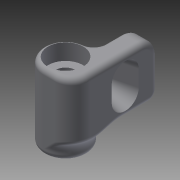
# Autodesk Inventor part: guia.tractora
Saved by Autodesk Inventor 2015 SP1 (Build 190203100, 203)
## iProperties
Created: 2015-07-01
Part Number: guia.tractora
Material: Generic
Document SubType Name: Modeling
Designer: pc
Density: 1 g/cm^3
Appearance: Default
Author: pc
Autodesk Inventor part; units mm, degrees
ref_plane "YZ Plane" through (0, 0, 0) normal (1, 0, 0) x (0, 1, 0)
ref_plane "XZ Plane" through (0, 0, 0) normal (0, 1, 0) x (-1, 0, 0)
ref_plane "XY Plane" through (0, 0, 0) normal (0, 0, 1) x (1, 0, 0)
sketch "Sketch10" plane through (0, 0, 0) normal (0, 0, 1) x (1, 0, 0)
  arc A0 (1.25, 3.7997) -> (0, -4) centre (0, 0) ccw
  line L0 (1.25, 3.7997) -> (1.25, 11.7997)
  line L1 (1.25, 11.7997) -> (5.25, 11.7997)
  line L2 (5.25, 11.7997) -> (5.25, -4)
  line L3 (5.25, -4) -> (0, -4)
  point P0 (1.25, -4)
  point P1 (1.25, -3)
  point P2 (3.25, 11.7997)
  dimension "d51" = 8
  dimension "d52" = 8
  dimension "d53" = 4
  dimension "d56" = 1.25
  constraints: 8 end point, 3 point on line, 2 perpendicular, 2 point on circle, 1 centre point, 1 coincident, 1 midpoint, 1 parallel, 1 tangent, 1 vertical
  measures "d51" diameter of A0
  measures "d52" distance of L0.start L0.end
  measures "d53" distance of L0.end L1.end
  measures "d56" distance from line of L0 point (0, 0)
extrude "Extrusion7" add sketch "Sketch10" along normal blind 10
sketch "Sketch15" plane through (0, 0, 0) normal (0, 0, -1) x (-1, 0, 0)
  arc A0 (0, -4) -> (-1.25, 3.7997) centre (0, 0) ccw projected
  circle A1 centre (0, 0) radius 4
  constraints: 1 centre point, 1 coincident, 1 concentric
extrude "Extrusion12" add sketch "Sketch15" along normal blind 4
sketch "Sketch16" plane through (0, 0, 10) normal (0, 0, 1) x (1, 0, 0)
  arc A0 (1.25, 3.7997) -> (0, -4) centre (0, 0) ccw projected
  circle A1 centre (0, 0) radius 3.25
  dimension "d71" = 6.5
  constraints: 1 centre point, 1 coincident
  measures "d71" diameter of A1
extrude "Extrusion13" cut sketch "Sketch16" against normal blind 3
sketch "Sketch17" plane through (0, 0, 7) normal (0, 0, 1) x (1, 0, 0)
  circle A0 centre (0, 0) radius 3.25 projected
  circle A1 centre (0, 0) radius 1.75
  dimension "d74" = 3.5
  constraints: 1 centre point, 1 coincident
  measures "d74" diameter of A1
extrude "Extrusion14" cut sketch "Sketch17" against normal through all contours A1
sketch "Sketch18" plane through (1.25, 3.7997, 0) normal (-1, 0, 0) x (0, 0, 1)
  line L0 (0, 8) -> (0, 0) projected
  line L1 (0, 0) -> (10, 0) projected
  line L2 (10, 8) -> (10, 0) projected
  line L3 (0, 8) -> (10, 8) projected
  line L4 (3.5, 2) -> (6.5, 2) construction
  line L5 (3.5, 0.5) -> (6.5, 0.5)
  line L6 (6.5, 3.5) -> (3.5, 3.5)
  arc A0 (3.5, 3.5) -> (3.5, 0.5) centre (3.5, 2) ccw
  arc A1 (6.5, 0.5) -> (6.5, 3.5) centre (6.5, 2) ccw
  point P0 (0, -3.7997)
  point P1 (5, 2)
  dimension "d77" = 3
  dimension "d78" = 3
  dimension "d79" = 6
  dimension "d80" = 5
  constraints: 8 end point, 4 point on circle, 4 tangent, 2 centre point, 1 horizontal, 1 midpoint, 1 parallel
  measures "d77" distance of L4.start L4.end
  measures "d78" diameter of A1
  measures "d79" distance from line of L3 point (5, 2)
  measures "d80" distance from line of L0 point (5, 2)
sketch "Sketch19" plane through (5.25, -4, 0) normal (1, 0, 0) x (0, 0, -1)
  line L0 (-10, 0) -> (-10, 15.7997) projected
  line L1 (0, 0) -> (0, 15.7997) projected
  line L2 (0, 15.7997) -> (-10, 15.7997) projected
  line L3 (-10, 0) -> (-10, 15.7997) projected
  line L4 (0, 0) -> (-10, 0) projected
  line L5 (0, 0) -> (-10, 0) projected
  line L6 (-10, 0) -> (-10, 15.7997) projected
  line L7 (-10, 15.7997) -> (0, 15.7997) projected
  line L8 (0, 15.7997) -> (0, 0) projected
  line L9 (0, 0) -> (-10, 0) projected
  line L10 (-10, 0) -> (-10, 15.7997) projected
  line L11 (-10, 15.7997) -> (0, 15.7997) projected
  line L12 (0, 15.7997) -> (0, 0) projected
  line L13 (-6.5, 11.2997) -> (-3.5, 11.2997) projected
  arc A0 (-6.5, 11.2997) -> (-6.5, 8.2997) centre (-6.5, 9.7997) ccw projected
  line L14 (-3.5, 8.2997) -> (-6.5, 8.2997) projected
  arc A1 (-3.5, 8.2997) -> (-3.5, 11.2997) centre (-3.5, 9.7997) ccw projected
  arc A2 (-6.5, 12.2997) -> (-6.5, 7.2997) centre (-6.5, 9.7997) ccw
  line L15 (-6.5, 12.2997) -> (-3.5, 12.2997)
  arc A3 (-3.5, 7.2997) -> (-3.5, 12.2997) centre (-3.5, 9.7997) ccw
  line L16 (-3.5, 7.2997) -> (-6.5, 7.2997)
  point P0 (0, 4)
  dimension "d90" = 1
  constraints: 4 end point, 4 point on circle, 2 centre point, 3 other
  measures "d90" radial gap between concentric circles of A0 A2
loft "Loft4" cut profiles "Sketch19", "Sketch18" contours L13 A1 L14 A0 | L15 A3 L16 A2 / A0 L6 A1 L5
fillet "Fillet5" radius 2.76 1 edges at (3.9496, -0.633, 0)
fillet "Fillet6" radius 2 2 edges at (1.25, 3.7997, 5) (1.25, 3.7997, -1.38)
fillet "Fillet7" radius 1.47 1 edges at (3.25, 11.7997, 0)
fillet "Fillet8" radius 2.81 1 edges at (3.25, 11.7997, 10)
fillet "Fillet9" radius 3.26 1 edges at (5.25, -4, 4.9977)
fillet "Fillet10" radius 1 20 edges at (5.25, 10.9766, 9.177) (5.25, 4.1248, 10) (4.2952, -3.0452, 10) (0.995, -4, 10) (-3.9921, -0.2505, 10) (0.75, 4.6301, 10) (1.25, 7.4713, 10) (1.25, 10.9766, 9.177) (1.25, 11.7997, 4.33) (1.25, 11.3691, 0.4306) (1.25, 8.4865, 0) (1.25, 6.2956, -0.0212) (0.4041, 4.3195, -1.4359) (5.25, 11.3691, 0.4306) (5.25, 7.2941, 0) (5.25, 1.7733, -0.2836) (4.2009, -3.1357, -0.4548) (1.6157, -4, -1.4815) (0.6194, -4, -2.2492) (5.25, 11.7997, 4.33)
fillet "Fillet11" radius 1 1 edges at (4, 0, -4)
body "Solid3"
